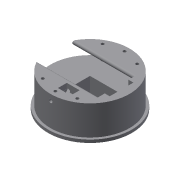
# Autodesk Inventor part: arm_0_top
Saved by Autodesk Inventor 2018 (Build 220112000, 112)
## iProperties
Created: 2017-12-03
Part Number: arm_0_top
Material: Generic
Document SubType Name: Modeling
Designer: Bardo91
Density: 1 g/cm^3
Appearance: Default
Mass: 106.152 g
Surface Area: 239.439 cm^2
Volume: 106.152 cm^3
Author: Bardo91
Autodesk Inventor part; units mm, degrees
ref_plane "YZ Plane" through (0, 0, 0) normal (1, 0, 0) x (0, 1, 0)
ref_plane "XZ Plane" through (0, 0, 0) normal (0, 1, 0) x (-1, 0, 0)
ref_plane "XY Plane" through (0, 0, 0) normal (0, 0, 1) x (1, 0, 0)
sketch "Sketch1" plane through (0, 0, 0) normal (0, 0, 1) x (1, 0, 0)
  circle A0 centre (0, 0) radius 40
  dimension "d0" = 80
  constraints: 1 centre point, 1 coincident
  measures "d0" diameter of A0
extrude "base" add sketch "Sketch1" along normal blind 30
sketch "Sketch3" plane through (0, 0, 0) normal (1, 0, 0) x (0, 1, 0)
  line L0 (40, 30) -> (-40, 30) projected
  line L1 (0, 30) -> (-15, 30)
  line L2 (0, 30) -> (15, 30)
  line L3 (15, 30) -> (29.1421, 15.8579)
  line L4 (-15, 30) -> (-29.1421, 15.8579)
  line L5 (-15, 30) -> (5, 30) construction
  line L6 (-29.1421, 15.8579) -> (29.1421, 15.8579)
  point P0 (0, 0)
  dimension "d13" = 15
  dimension "d14" = 15
  dimension "d15" = 20
  dimension "d16" = 135
  dimension "d17" = 20
  dimension "d18" = 135
  constraints: 12 end point, 2 point on line, 1 equal length, 1 horizontal, 1 midpoint
  measures "d13" distance of L1.start L1.end
  measures "d14" distance of L1.start L2.end
  measures "d15" distance of L2.end L3.end
  measures "d16" angle of L2 L3
  measures "d17" distance of L1.end L4.end
  measures "d18" angle of L4 L5
extrude "horse_tail_1" cut sketch "Sketch3" against normal up to surface round surface about axis through (0, 0, 0) along (0, 0, 1) radius 40 far side no
mirror "horse_tail_2" about plane through (0, 0, 21.3699) normal (-1, 0, 0) of "horse_tail_1"
fillet "fillet_horse_tail" radius 2 2 edges at (0, 15, 30) (0, -15, 30)
sketch "Sketch4" plane through (0, 0, 0) normal (0, 1, 0) x (-1, 0, 0)
  line L0 (34.7395, 30) -> (-34.7395, 30) projected
  circle A0 centre (0, 23.8579) radius 1.75
  line L1 (0, 23.8579) -> (0, 15.8579)
  line L2 (-27.3996, 15.8579) -> (27.3996, 15.8579) projected
  point P0 (0, 0)
  dimension "d20" = 3.5
  dimension "d23" = 8
  constraints: 2 end point, 1 centre point, 1 midpoint
  measures "d20" diameter of A0
  measures "d23" distance of L1.start L1.end
extrude "lock_arm" cut sketch "Sketch4" along normal through all both and the other way through all
sketch "Sketch5" plane through (-27.3996, -29.1421, 15.8579) normal (0, 0, 1) x (1, 0, 0)
  line L0 (27.3996, 29.1421) -> (27.3996, 19.1421)
  line L1 (27.3996, 19.1421) -> (17.3996, 19.1421)
  line L2 (17.3996, 19.1421) -> (17.3996, 39.1421)
  line L3 (17.3996, 39.1421) -> (57.3996, 39.1421)
  line L4 (57.3996, 39.1421) -> (57.3996, 19.1421)
  line L5 (57.3996, 19.1421) -> (27.3996, 19.1421)
  dimension "d24" = 10
  dimension "d25" = 10
  dimension "d26" = 20
  dimension "d27" = 40
  constraints: 12 end point, 5 perpendicular, 1 point on line, 1 vertical
  measures "d24" distance of L0.start L0.end
  measures "d25" distance of L0.end L1.end
  measures "d26" distance of L1.end L2.end
  measures "d27" distance of L2.end L3.end
extrude "servo_place" cut sketch "Sketch5" against normal through all
sketch "Sketch6" plane through (0, 0, 0) normal (0, 0, -1) x (-1, 0, 0)
  circle A0 centre (0, 0) radius 10
  circle A1 centre (0, 0) radius 42.5
  dimension "d30" = 20
  dimension "d31" = 85
  constraints: 2 centre point, 2 coincident
  measures "d30" diameter of A0
  measures "d31" diameter of A1
extrude "base_hold" add sketch "Sketch6" along normal blind 3
sketch "Sketch7" plane through (-27.3996, -29.1421, 15.8579) normal (0, 0, 1) x (1, 0, 0)
  arc A0 (54.3996, -0.3706) -> (54.3996, 58.6548) centre (27.3996, 29.1421) ccw
  line L0 (27.3996, 29.1421) -> (67.3996, 29.1421)
  line L1 (67.3996, 29.1421) -> (59.3996, 29.1421)
  line L2 (59.3996, 29.1421) -> (59.3996, 17.1421)
  line L3 (59.3996, 29.1421) -> (59.3996, 41.1421)
  line L4 (59.3996, 41.1421) -> (54.3996, 41.1421)
  line L5 (54.3996, 41.1421) -> (54.3996, 58.6548)
  arc A1 (62.1391, 48.9706) -> (-7.3399, 48.9706) centre (27.3996, 29.1421) ccw projected
  line L6 (59.3996, 17.1421) -> (54.3996, 17.1421)
  line L7 (54.3996, 17.1421) -> (54.3996, -0.3706)
  dimension "d34" = 8
  dimension "d35" = 12
  dimension "d36" = 12
  dimension "d37" = 5
  dimension "d38" = 5
  constraints: 16 end point, 4 perpendicular, 4 point on circle, 3 point on line, 1 centre point, 1 coincident, 1 horizontal
  measures "d34" distance of L0.end L1.end
  measures "d35" distance of L1.end L2.end
  measures "d36" distance of L1.end L3.end
  measures "d37" distance of L3.end L4.end
  measures "d38" distance of L2.end L6.end
extrude "horse_tal_end" add sketch "Sketch7" along normal up to surface (14.1421 mm away)
sketch "Sketch8" plane through (0, 0, 30) normal (0, 0, 1) x (1, 0, 0)
  circle A0 centre (0, 0) radius 35
  line L0 (0, -35) -> (0, 35)
  line L1 (-17.5, -30.3109) -> (17.5, 30.3109)
  line L2 (0, 0) -> (35, 0) construction
  line L3 (17.5, -30.3109) -> (-17.5, 30.3109)
  line L4 (0, 0) -> (35, 0) construction
  circle A1 centre (17.5, -30.3109) radius 1.5
  circle A2 centre (0, -35) radius 1.5
  circle A3 centre (-17.5, -30.3109) radius 1.5
  circle A4 centre (-17.5, 30.3109) radius 1.5
  circle A5 centre (0, 35) radius 1.5
  circle A6 centre (17.5, 30.3109) radius 1.5
  dimension "d41" = 70
  dimension "d42" = 60
  dimension "d43" = 120
  dimension "d44" = 3
  dimension "d45" = 3
  dimension "d46" = 3
  dimension "d47" = 3
  dimension "d48" = 3
  dimension "d49" = 3
  constraints: 10 end point, 6 centre point, 6 coincident, 3 midpoint, 2 horizontal, 1 vertical, 9 other
  measures "d42" angle of L2 L1
  measures "d43" angle of L4 L3
  measures "d44" diameter of A1
  measures "d45" diameter of A2
  measures "d46" diameter of A3
  measures "d47" diameter of A4
  measures "d48" diameter of A5
  measures "d49" diameter of A6
extrude "reinforcement_holes" cut sketch "Sketch8" against normal through all contours A6 L1 A0 | A0 A6 | A1 A0 | A0 L3 A1 | L1 A6 A0 | A0 A1 L3 | A5 L0 A0 | A0 A5 | A2 A0 L0 | L0 A0 A2 | A5 A0 L0 | A3 A0 L1 | L1 A0 A3 | A4 A0 L3 | L3 A0 A4 | A2 A0 | A0 A3 | A0 A4
sketch "Sketch9" plane through (0, 0, 30) normal (0, 0, 1) x (1, 0, 0)
  line L0 (27, 19.8284) -> (-34.7395, 19.8284) projected
  line L1 (0, 0) -> (0, -22)
  line L2 (0, -22) -> (5, -22)
  line L3 (5, -22) -> (11.5, -22)
  line L4 (11.5, -22) -> (11.5, -31)
  line L5 (11.5, -31) -> (-1.5, -31)
  line L6 (-1.5, -31) -> (-1.5, -22)
  line L7 (-1.5, -31) -> (7.5, -31) construction
  line L8 (-1.5, -22) -> (0, -22)
  dimension "d62" = 22
  dimension "d63" = 5
  dimension "d64" = 6.5
  dimension "d65" = 9
  dimension "d66" = 13
  dimension "d67" = 9
  dimension "d68" = 90
  constraints: 16 end point, 4 perpendicular, 2 vertical, 1 horizontal, 1 point on line
  measures "d62" distance of L1.start L1.end
  measures "d63" distance of L1.end L2.end
  measures "d64" distance of L2.end L3.end
  measures "d65" distance of L3.end L4.end
  measures "d66" distance of L4.end L5.end
  measures "d67" distance of L5.end L6.end
  measures "d68" angle of L7 L6
extrude "cable_hole" cut sketch "Sketch9" against normal through all
sketch "Sketch10" plane through (0, 0, -3) normal (0, 0, -1) x (-1, 0, 0)
  line L0 (1.5, -31) -> (-11.5, -31) projected
  arc A0 (-27.0847, -18.9649) -> (27.0847, -18.9649) centre (0, 0) ccw
  line L1 (0, 0) -> (-27.0847, -18.9649)
  line L2 (0, 0) -> (33.0643, 0) construction
  line L3 (0, 0) -> (27.0847, -18.9649)
  arc A1 (-16.383, -11.4715) -> (16.383, -11.4715) centre (0, 0) ccw
  point P0 (17.4871, -12.2446)
  point P1 (-17.4871, -12.2446)
  dimension "d69" = 145
  dimension "d74" = 40
  constraints: 6 end point, 5 point on circle, 4 point on line, 3 coincident, 2 centre point, 1 equal length, 1 horizontal
  measures "d69" angle of L1 L2
  measures "d74" diameter of A1
extrude "Extrusion10" cut sketch "Sketch10" against normal blind 5 contours L1 A1 L3 A0
fillet "Fillet3" radius 5 4 edges at (0, -33.0643, -3) (-21.7339, -15.2182, -3) (0, -20, -3) (21.7339, -15.2182, -3)
body "Solid1"
